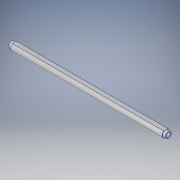
# Autodesk Inventor part: Belt Axle
Saved by Autodesk Inventor 2019.4 (Build 234330000, 330)
## iProperties
Created: 2020-01-11
Part Number: Belt Axle
Material: Aluminum 6061
Document SubType Name: Modeling
Designer: admin
Density: 2.7 g/cm^3
Appearance: Aluminum - Flat
Mass: 50.0907 g
Surface Area: 137.201 cm^2
Volume: 18.5521 cm^3
Author: admin
Autodesk Inventor part; units mm, degrees
ref_plane "YZ Plane" through (0, 0, 0) normal (1, 0, 0) x (0, 1, 0)
ref_plane "XZ Plane" through (0, 0, 0) normal (0, 1, 0) x (-1, 0, 0)
ref_plane "XY Plane" through (0, 0, 0) normal (0, 0, 1) x (1, 0, 0)
sketch "Sketch1" plane through (0, 0, 0) normal (0, 0, 1) x (1, 0, 0)
  line L0 (0, 0) -> (0, 4.9)
  line L1 (0, 4.9) -> (4, 4.9)
  line L2 (4, 4.9) -> (4, 5.9)
  line L3 (4, 5.9) -> (241.2, 5.9)
  line L4 (241.2, 5.9) -> (241.2, 4.9)
  line L5 (241.2, 4.9) -> (245.2, 4.9)
  line L6 (245.2, 4.9) -> (245.2, 0)
  line L7 (245.2, 0) -> (0, 0)
  dimension "d0" = 4.9
  dimension "d1" = 5.9
  dimension "d2" = 4
  dimension "d3" = 237.2
  dimension "d4" = 4
  constraints: 16 end point, 6 perpendicular, 2 point on line, 1 vertical
  measures "d0" distance between parallel lines of L7 L1
  measures "d1" distance between parallel lines of L7 L3
  measures "d2" distance of L4.end L5.end
  measures "d3" distance of L2.end L3.end
  measures "d4" distance of L0.end L1.end
revolve "Revolution1" add sketch "Sketch1" angle 360 about axis through (245.2, 0, 0) along (-1, 0, 0)
sketch "Sketch2" plane through (241.2, 0, 0) normal (1, 0, 0) x (0, 0, -1)
  circle A0 centre (0, 0) radius 5.9 projected
  line L0 (-3.2863, 4.9) -> (3.2863, 4.9)
  circle A1 centre (0, 0) radius 4.9 projected
  constraints: 2 end point, 2 point on circle, 1 horizontal, 1 tangent
extrude "Extrusion1" cut sketch "Sketch2" against normal through all contours L0 A0 picked at (1.778, 5.1111)
sketch "Sketch3" plane through (245.2, 0, 0) normal (1, 0, 0) x (0, 0, -1)
  circle A0 centre (0, 0) radius 4.9 projected
  constraints: 1 coincident
hole "Hole1" at (245.2, 0, 0) direction (-1, 0, 0) diameter 6 end through all
body "Solid1"
